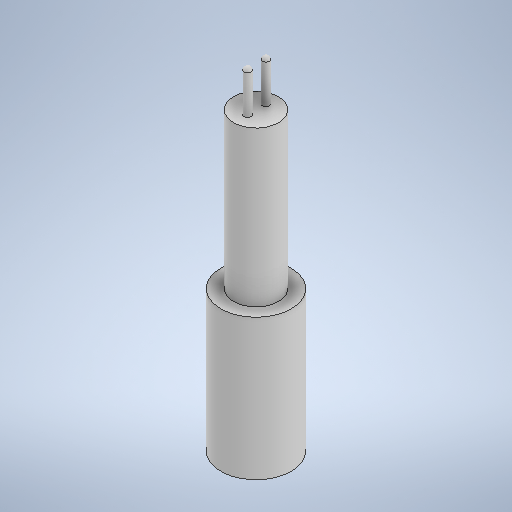
# Autodesk Inventor part: Arc Water Sensor
Saved by Autodesk Inventor 2025 (Build 290162000, 162)
## iProperties
Created: 2024-07-09
Part Number: Arc Water Sensor
Material: Generic
Document SubType Name: Modeling
Designer: track
Density: 1 g/cm^3
Appearance: Default
Author: track
Autodesk Inventor part; units mm, degrees
ref_plane "YZ Plane" through (0, 0, 0) normal (1, 0, 0) x (0, 1, 0)
ref_plane "XZ Plane" through (0, 0, 0) normal (0, 1, 0) x (-1, 0, 0)
ref_plane "XY Plane" through (0, 0, 0) normal (0, 0, 1) x (1, 0, 0)
sketch "Sketch1" plane through (0, 0, 0) normal (0, 1, 0) x (-1, 0, 0)
  circle A0 centre (0, 0) radius 3.2
  dimension "d0" = 6.4
  constraints: 1 centre point, 1 coincident
  measures "d0" diameter of A0
extrude "Extrusion1" add sketch "Sketch1" against normal blind 42
sketch "Sketch2" plane through (0, -42, 0) normal (0, -1, 0) x (1, 0, 0)
  circle A0 centre (0, 0) radius 5
  dimension "d3" = 10
  constraints: 1 centre point, 1 coincident
  measures "d3" diameter of A0
extrude "Extrusion2" add sketch "Sketch2" against normal blind 20
sketch "Sketch3" plane through (0, 0, 0) normal (0, 1, 0) x (1, 0, 0)
  circle A0 centre (0, 0) radius 3.2 projected
  line L0 (0, -3.2) -> (0, 3.2) construction
  circle A1 centre (0, -1.2) radius 0.5
  circle A2 centre (0, 1.4) radius 0.5
  dimension "d6" = 0
  dimension "d7" = 1
  dimension "d8" = 1
  dimension "d9" = 1.8
  dimension "d10" = 2.6
  constraints: 2 centre point, 2 end point, 2 point on circle, 2 point on line, 1 vertical
  measures "d6" distance from line of point (0, 0) L0
  measures "d7" diameter of A2
  measures "d8" diameter of A1
  measures "d9" distance of L0.end A2.centre
  measures "d10" distance of A1.centre A2.centre
extrude "Extrusion3" add sketch "Sketch3" along normal blind 6 contours A1 | A2
fillet "Fillet1" radius 0.5 2 edges at (-0.5, 6, -1.4) (-0.5, 6, 1.2)
body "Solid1"
